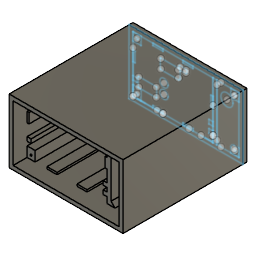
DD-boitier-V6 (Autodesk Fusion 360 design; units mm, degrees)
part number: 2025-12-19-14-32-53-043
Autodesk Fusion 360 part; units mm, degrees
note: some values were not read from the file. Set by a fixed rule: which sketch regions a step uses.
sketch "Esquisse1" plane through (0, 0, 0) normal (0, 1, 0) x (1, 0, 0)
  line L0 (0, -28) -> (40, -28)
  line L1 (40, -28) -> (40, 0)
  line L2 (40, 0) -> (42, 0)
  line L3 (42, 0) -> (42, -28)
  line L4 (42, -28) -> (40, -28)
  line L5 (40, -28) -> (40, 0)
  line L6 (42, 0) -> (53, 0)
  line L7 (53, 0) -> (53, -28)
  line L8 (53, -28) -> (42, -28)
  line L9 (42, -28) -> (42, 0)
  line L10 (12, 0) -> (15, 0)
  line L11 (25, 0) -> (28, 0)
  line L12 (10, -28) -> (15, -28)
  line L13 (15, -28) -> (15, -27)
  line L14 (15, -27) -> (10, -27)
  line L15 (10, -27) -> (10, -28)
  line L16 (30, -28) -> (25, -28)
  line L17 (25, -28) -> (25, -27)
  line L18 (25, -27) -> (30, -27)
  line L19 (30, -27) -> (30, -28)
  line L20 (0, -5) -> (0, -3)
  line L21 (40, -5) -> (40, -3)
  line L22 (40, -7) -> (38, -7)
  line L23 (38, -7) -> (38, -9)
  line L24 (38, -9) -> (40, -9)
  line L25 (40, -9) -> (40, -7)
  line L26 (2.8548, -5.1537) -> (11.6265, -5.1537)
  line L27 (11.8666, -5.3938) -> (11.8666, -9.7641)
  line L28 (11.6265, -10.0042) -> (2.8548, -10.0042)
  line L29 (2.6148, -9.7641) -> (2.6148, -5.3938)
  circle A0 centre (15.5, -8.5) radius 2
  circle A1 centre (15.5, -13.5) radius 2
  line L30 (0, 0) -> (40, 0)
  line L31 (0, 0) -> (0, -28)
  line L32 (0, -7) -> (2, -7)
  line L33 (2, -7) -> (2, -9)
  line L34 (2, -9) -> (0, -9)
  line L35 (0, -9) -> (0, -7)
  line L36 (-2, -30) -> (55, -30)
  line L37 (55, -30) -> (55, 2)
  line L38 (55, 2) -> (-2, 2)
  line L39 (-2, 2) -> (-2, -30)
  line L40 (0, 0) -> (15, 0)
  line L41 (13.9, -18.5) -> (22.7767, -18.5)
  line L42 (23.531, -19.2543) -> (23.531, -22.7696)
  line L43 (22.7767, -23.5239) -> (13.9, -23.5239)
  line L44 (13.66, -23.2839) -> (13.66, -18.7401)
  line L45 (0, -20) -> (1, -20)
  line L46 (1, -20) -> (1, -15)
  line L47 (1, -15) -> (0, -15)
  line L48 (0, -15) -> (0, -20)
  line L49 (40, -16) -> (40, -20)
  line L50 (44, -28) -> (42, -26)
  line L51 (44, 0) -> (42, -2)
  line L52 (10, 0) -> (15, 0)
  line L53 (15, 0) -> (15, -1)
  line L54 (15, -1) -> (10, -1)
  line L55 (10, -1) -> (10, 0)
  line L56 (25, 0) -> (30, 0)
  line L57 (30, 0) -> (30, -1)
  line L58 (30, -1) -> (25, -1)
  line L59 (25, -1) -> (25, 0)
  line L60 (40, -20) -> (39, -20)
  line L61 (39, -20) -> (39, -15)
  line L62 (39, -15) -> (40, -15)
  line L63 (40, -15) -> (40, -20)
  line L64 (0, -21) -> (0, 0)
  line L65 (27, -23.5239) -> (27, -24.5)
  line L66 (26.5, -25) -> (23.5232, -25)
  arc A2 (11.6265, -10.0042) -> (11.8666, -9.7641) centre (11.6265, -9.7641) ccw
  arc A3 (2.6148, -9.7641) -> (2.8548, -10.0042) centre (2.8548, -9.7641) ccw
  arc A4 (2.8548, -5.1537) -> (2.6148, -5.3938) centre (2.8548, -5.3938) ccw
  arc A5 (11.8666, -5.3938) -> (11.6265, -5.1537) centre (11.6265, -5.3938) ccw
  arc A6 (13.9, -18.5) -> (13.66, -18.7401) centre (13.9, -18.7401) ccw
  arc A7 (13.66, -23.2839) -> (13.9, -23.5239) centre (13.9, -23.2839) ccw
  arc A8 (23.531, -19.2543) -> (22.7767, -18.5) centre (22.7767, -19.2543) ccw
  arc A9 (22.7767, -23.5239) -> (23.531, -22.7696) centre (22.7767, -22.7696) ccw
  line L67 (26.5, -23.0239) -> (23.6, -23.0239)
  line L68 (23, -23.6) -> (23.0141, -24.4988)
  arc A10 (27, -23.5239) -> (26.5, -23.0239) centre (26.5, -23.5239) ccw
  arc A11 (26.5, -25) -> (27, -24.5) centre (26.5, -24.5) ccw
  arc A12 (23.0141, -24.4988) -> (23.5232, -25) centre (23.5232, -24.4909) ccw
  line L69 (6, 0) -> (0, 0)
  line L70 (0, 0) -> (0, -3)
  line L71 (40, -3) -> (40, 0)
  line L72 (40, 0) -> (34, 0)
  line L73 (0, -28) -> (4, -28)
  line L74 (4, -28) -> (4, -24)
  line L75 (4, -24) -> (0, -24)
  line L76 (0, -24) -> (0, -28)
  line L77 (49, -28) -> (53, -28)
  line L78 (53, -28) -> (53, -24)
  line L79 (53, -24) -> (50.5, -24)
  line L80 (49, -25.5) -> (49, -28)
  line L81 (53, 0) -> (49, 0)
  line L82 (49, 0) -> (49, -2.5)
  line L83 (50.5, -4) -> (53, -4)
  line L84 (53, -4) -> (53, 0)
  line L85 (0, -5) -> (4, -5)
  line L86 (4, -5) -> (4, 0)
  line L87 (4, 0) -> (0, 0)
  line L88 (0, 0) -> (0, -5)
  line L89 (36, 0) -> (40, 0)
  line L90 (40, 0) -> (40, -5)
  line L91 (40, -5) -> (38, -5)
  line L92 (38, -5) -> (38, -3)
  line L93 (38, -3) -> (40, -3)
  line L94 (40, -3) -> (40, -5)
  circle A13 centre (2, -26) radius 0.5
  circle A14 centre (2, -2) radius 0.5
  circle A15 centre (51, -2) radius 0.5
  circle A16 centre (51, -26) radius 0.5
  arc A17 (50.5, -24) -> (49, -25.5) centre (50.5, -25.5) ccw
  arc A18 (49, -2.5) -> (50.5, -4) centre (50.5, -2.5) ccw
  circle A19 centre (47, -22) radius 3
  line L95 (23, -23.6) -> (23.6, -23.0239)
  dimension "d131" = 1
  dimension "d132" = 1
  dimension "d133" = 1
  dimension "d134" = 1
  dimension "d136" = 1.5
  dimension "d160" = 6
  constraint horizontal L0
  constraint vertical L1
  constraint horizontal L2
  constraint vertical L3
  constraint horizontal L4
  constraint vertical L5
  constraint horizontal L6
  constraint vertical L7
  constraint horizontal L8
  constraint vertical L9
  constraint horizontal L10
  constraint horizontal L11
  constraint horizontal L12
  constraint vertical L13
  constraint horizontal L14
  constraint vertical L15
  constraint horizontal L16
  constraint vertical L17
  constraint horizontal L18
  constraint vertical L19
  constraint vertical L20
  constraint vertical L21
  constraint horizontal L22
  constraint vertical L23
  constraint horizontal L24
  constraint vertical L25
  constraint horizontal L26
  constraint vertical L27
  constraint horizontal L28
  constraint vertical L29
  constraint perpendicular L1 L30
  constraint perpendicular L0 L31
  constraint horizontal L32
  constraint vertical L33
  constraint horizontal L34
  constraint vertical L35
  constraint horizontal L36
  constraint vertical L37
  constraint horizontal L38
  constraint vertical L39
  constraint horizontal L40
  constraint horizontal L41
  constraint vertical L42
  constraint horizontal L43
  constraint vertical L44
  constraint horizontal L45
  constraint vertical L46
  constraint horizontal L47
  constraint vertical L48
  constraint vertical L49
  constraint horizontal L52
  constraint vertical L53
  constraint horizontal L54
  constraint vertical L55
  constraint horizontal L56
  constraint vertical L57
  constraint horizontal L58
  constraint vertical L59
  constraint horizontal L60
  constraint vertical L61
  constraint horizontal L62
  constraint vertical L63
  constraint vertical L64
  constraint vertical L65
  constraint horizontal L66
  constraint tangent L27 A2
  constraint tangent L28 A2
  constraint tangent L28 A3
  constraint tangent L29 A3
  constraint equal A2 A3
  constraint tangent L26 A4
  constraint tangent L29 A4
  constraint equal A2 A4
  constraint tangent L26 A5
  constraint tangent L27 A5
  constraint equal A2 A5
  constraint tangent L41 A6
  constraint tangent L44 A6
  constraint equal A2 A6
  constraint tangent L43 A7
  constraint tangent L44 A7
  constraint equal A2 A7
  constraint tangent L41 A8
  constraint tangent L42 A8
  constraint tangent L42 A9
  constraint tangent L43 A9
  constraint equal A8 A9
  constraint perpendicular L65 L67
  constraint tangent L65 A10
  constraint tangent L67 A10
  constraint tangent L65 A11
  constraint tangent L66 A11
  constraint tangent L66 A12
  constraint tangent L68 A12
  constraint horizontal L69
  constraint vertical L70
  constraint coincident L40 L69.start
  constraint vertical L71
  constraint horizontal L72
  constraint horizontal L73
  constraint vertical L74
  constraint horizontal L75
  constraint vertical L76
  constraint horizontal L77
  constraint vertical L78
  constraint horizontal L79
  constraint vertical L80
  constraint coincident L7 L78.end
  constraint horizontal L81
  constraint vertical L82
  constraint horizontal L83
  constraint vertical L84
  constraint horizontal L85
  constraint vertical L86
  constraint horizontal L87
  constraint vertical L88
  constraint coincident L69 L86.end
  constraint horizontal L89
  constraint vertical L90
  constraint coincident L72 L89.start
  constraint horizontal L91
  constraint vertical L92
  constraint horizontal L93
  constraint vertical L94
  constraint tangent L79 A17
  constraint tangent L80 A17
  constraint tangent L82 A18
  constraint tangent L83 A18
  measures "d131" diameter of A13
  measures "d132" diameter of A14
  measures "d133" diameter of A15
  measures "d134" diameter of A16
  measures "d136" radius of A18
  measures "d160" diameter of A19
extrude "Extrusion35" add sketch "Esquisse1" along normal blind 2 contours L0 L31 L73 L74 L75 L76 | L0 L1 L5 L13 L14 L15 L17 L18 L19 L22 L23 L24 L30 L31 L32 L33 L34 L40 L45 L46 L47 L53 L54 L55 L57 L58 L59 L60 L61 L62 L64 L69 L71 L72 L74 L75 L85 L86 L89 L90 L91 L92 L93 | L0 L12 L13 L14 L15 | L31 L45 L46 L47 L48 L64 | L0 L16 L17 L18 L19 | L31 L32 L33 L34 L35 L64 | L1 L2 L3 L4 L5 L9 L21 L25 L49 L63 L71 L90 L94 | L1 L5 L49 L60 L61 L62 L63 | L3 L8 L9 L50 | L20 L30 L31 L40 L64 L69 L70 L85 L86 L87 L88 | L3 L6 L7 L8 L9 L50 L51 L79 L80 L82 L83 A17 A18 | L3 L6 L9 L51 | L7 L8 L77 L78 L79 L80 A17 | L1 L5 L22 L23 L24 L25 | L6 L7 L81 L82 L83 L84 A18 | L10 L30 L40 L52 L53 L54 L55 | L1 L5 L21 L90 L91 L92 L93 L94 | L11 L30 L56 L57 L58 L59 | L36 L37 L38 L39 | L65 L66 L67 L68 A10 A11 A12 L95 | A13 | A14 | A15 | A16 makes body 1
extrude "Extrusion36" add sketch "Esquisse1" against normal blind 53 separate body contours L0 L31 L73 L74 L75 L76 | L0 L12 L13 L14 L15 | L31 L45 L46 L47 L48 L64 | L0 L16 L17 L18 L19 | L31 L32 L33 L34 L35 L64 | L1 L2 L3 L4 L5 L9 L21 L25 L49 L63 L71 L90 L94 | L1 L5 L49 L60 L61 L62 L63 | L3 L8 L9 L50 | L20 L30 L31 L40 L64 L69 L70 L85 L86 L87 L88 | L3 L6 L9 L51 | L7 L8 L77 L78 L79 L80 A17 | L1 L5 L22 L23 L24 L25 | L6 L7 L81 L82 L83 L84 A18 | L10 L30 L40 L52 L53 L54 L55 | L1 L5 L21 L90 L91 L92 L93 L94 | L11 L30 L56 L57 L58 L59 makes body 2 at (13.3333, -17.6667, 27) makes body 3 at (11.6667, -17.6667, 0) makes body 4 at (2.6667, -35.3333, 24) makes body 5 at (0, -17.6667, 3.3333) makes body 6 at (26.6667, -17.6667, 27) makes body 7 at (53, -17.6667, 25.3333) makes body 8 at (28.3333, -17.6667, 1) makes body 9 at (0, -17.6667, 16.6667) makes body 10 at (0, -17.6667, 7.6667) makes body 11 at (42, -35.3333, 18) makes body 12 at (53, -17.6667, 1.3333)
extrude "Extrusion37" add sketch "Esquisse1" against normal blind 60 separate body contours L36 L37 L38 L39 makes body 13
extrude "Extrusion38" add sketch "Esquisse1" along normal blind 1 separate body contours L65 L66 L67 L68 A10 A11 A12 L95 makes body 14
extrude "Extrusion1" [suppressed]
extrude "Extrusion2" [suppressed]
extrude "Extrusion3" [suppressed]
